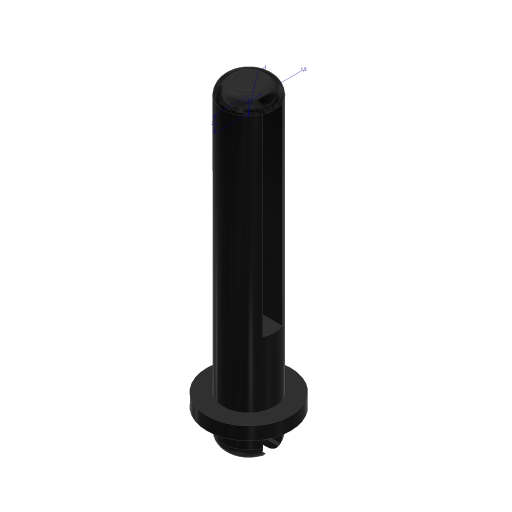
# Autodesk Inventor part: Federbalken
Saved by Autodesk Inventor 2023 (Build 270158000, 158)
## iProperties
Created: 2025-01-21
Part Number: Federbalken
Material: Acetalharz, Schwarz
Document SubType Name: Modeling
Designer: abdel
Density: 1.425 g/cm^3
Appearance: Glatt - Schwarz
Author: abdel
Autodesk Inventor part; units mm, degrees
ref_plane "YZ Plane" through (0, 0, 0) normal (1, 0, 0) x (0, 1, 0)
ref_plane "XZ Plane" through (0, 0, 0) normal (0, 1, 0) x (-1, 0, 0)
ref_plane "XY Plane" through (0, 0, 0) normal (0, 0, 1) x (1, 0, 0)
sketch "Skizze1" plane through (0, 0, 0) normal (0, 0, 1) x (1, 0, 0)
  circle A0 centre (0, 0) radius 4
  dimension "d1" = 8
  constraints: 1 centre point, 1 coincident
  measures "d1" diameter of A0
extrude "Extrusion1" add sketch "Skizze1" along normal blind 44
sketch "Skizze2" plane through (0, 0, 0) normal (1, 0, 0) x (0, 1, 0)
  line L0 (0, -10) -> (0, 60) projected
  line L1 (-5.6, 0) -> (5.6, 0) projected
  line L2 (4, 0) -> (4, 44) projected
  line L3 (4, 44) -> (-4, 44) projected
  line L4 (-4, 0) -> (-4, 44) projected
  line L5 (1.5, 42) -> (1.5, 12)
  line L6 (-1.5, 42) -> (-1.5, 12)
  line L7 (1.5, 42) -> (-1.5, 42)
  line L8 (1.5, 12) -> (-1.5, 12)
  point P0 (0, 0)
  dimension "d4" = 30
  dimension "d6" = 3
  dimension "d7" = 2
  constraints: 8 end point, 2 horizontal, 2 vertical, 1 parallel, 1 other
  measures "d4" distance of L5.start L5.end
  measures "d6" distance of L5.end L6.end
  measures "d7" distance between parallel lines of L7 L3
extrude "Extrusion2" cut sketch "Skizze2" along normal mid plane 40 contours L8 L6 L7 L0 | L0 L7 L5 L8
sketch "Skizze6" plane through (0, 0, 0) normal (0, 1, 0) x (-1, 0, 0)
  line L0 (4, 0) -> (4, 44) projected
  line L1 (4, 0) -> (-4, 0) projected
  line L2 (-4, 0) -> (-4, 44) projected
  line L3 (3.7081, 12) -> (-3.7081, 12) projected
  line L4 (-4, 12) -> (-3.7081, 12) projected
  line L5 (3.7081, 12) -> (4, 12) projected
  line L6 (6.5, 2) -> (4, 2)
  line L7 (4, 2) -> (4, 0)
  line L8 (4, 0) -> (6.5, 0)
  line L9 (6.5, 0) -> (6.5, 2)
  line L10 (0, -10) -> (0, 60) projected
  point P0 (0, 0)
  dimension "d22" = 2
  dimension "d23" = 2.5
  constraints: 8 end point, 2 parallel, 1 horizontal, 1 perpendicular
  measures "d22" distance of L8.end L6.start
  measures "d23" distance of L6.start L6.end
revolve "Umdrehung1" add sketch "Skizze6" angle 360 about axis through (0, 0, -10) along (0, 0, 1) contours L0 L6 L9 L8
sketch "Skizze7" plane through (0, 0, 0) normal (0, 0, -1) x (-1, 0, 0)
  circle A0 centre (0, 0) radius 4 projected
  circle A1 centre (0, 0) radius 4
  constraints: 1 centre point, 1 coincident, 1 concentric
extrude "Extrusion5" add sketch "Skizze7" along normal blind 5
sketch "Skizze8" plane through (0, 0, -5) normal (0, 0, -1) x (-1, 0, 0)
  circle A0 centre (0, 0) radius 4 projected
  line L0 (3.7081, -1.5) -> (-3.7081, -1.5)
  line L1 (3.7081, 1.5) -> (-3.7081, 1.5)
  dimension "d28" = 3
  constraints: 4 end point, 4 point on circle, 2 parallel, 1 horizontal
  measures "d28" distance between parallel lines of L1 L0
extrude "Extrusion6" cut sketch "Skizze8" against normal blind 3 contours A0 L0 L1
sketch "Skizze9" plane through (-3.7081, -1.5, -5) normal (0, 1, 0) x (1, 0, 0)
  line L0 (0, 0) -> (7.4162, 0) projected
  line L1 (0, -3) -> (0, 0) projected
  line L2 (7.4162, 0) -> (7.4162, -3) projected
  line L3 (0, 0) -> (7.4162, 0)
  line L4 (7.4162, 0) -> (7.4162, -1)
  line L5 (7.4162, -1) -> (0, -1)
  line L6 (0, -1) -> (0, 0)
  point P0 (3.7081, -5)
  point P1 (0, -1)
  dimension "d31" = 1
  constraints: 8 end point, 2 parallel, 1 horizontal, 1 perpendicular, 1 point on line
  measures "d31" distance between parallel lines of L5 L0
sketch "Skizze10" plane through (-3.7081, 1.5, -5) normal (0, -1, 0) x (1, 0, 0)
  line L0 (7.4162, 0) -> (0, 0) projected
  line L1 (7.4162, 3) -> (7.4162, 0) projected
  line L2 (0, 0) -> (0, 3) projected
  line L3 (0, 0) -> (7.4162, 0)
  line L4 (7.4162, 0) -> (7.4162, 1)
  line L5 (7.4162, 1) -> (0, 1)
  line L6 (0, 1) -> (0, 0)
  point P0 (3.7081, 5)
  dimension "d32" = 1
  constraints: 8 end point, 3 point on line, 2 parallel, 1 horizontal, 1 perpendicular
  measures "d32" distance between parallel lines of L5 L0
extrude "Extrusion7" add sketch "Skizze9" along normal blind 0.5
extrude "Extrusion8" add sketch "Skizze10" along normal blind 0.5
sketch "Skizze11" plane through (0, 0, 0) normal (1, 0, 0) x (0, 1, 0)
  circle A0 centre (0, 39.5) radius 0.5
  line L0 (1.5, 42) -> (-1.5, 42) projected
  line L1 (1.5, 12) -> (1.5, 42) projected
  point P0 (0, 0)
  point P1 (0, 42)
  dimension "d37" = 1
  dimension "d38" = 2.5
  dimension "d39" = 1.5
  constraints: 1 centre point, 1 midpoint
  measures "d37" diameter of A0
  measures "d38" distance of point (0, 42) A0.centre
  measures "d39" distance from line of L1 A0.centre
fillet "Rundung4" radius 2 3 edges at (-4, 0, 44) (0, 4, -5) (0, -4, -5)
